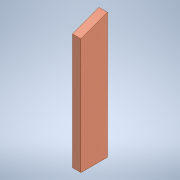
# Autodesk Inventor part: 2x6SupportBracket
Saved by Autodesk Inventor 2022.2 (Build 262287000, 287)
## iProperties
Created: 2021-11-26
Part Number: 2x6SupportBracket
Material: Wood (Walnut)
Document SubType Name: Modeling
Designer: robst
Density: 0.55 g/cm^3
Appearance: Walnut - Natural Polished
Author: robst
Autodesk Inventor part; units mm, degrees
ref_plane "YZ Plane" through (0, 0, 0) normal (1, 0, 0) x (0, 1, 0)
ref_plane "XZ Plane" through (0, 0, 0) normal (0, 1, 0) x (-1, 0, 0)
ref_plane "XY Plane" through (0, 0, 0) normal (0, 0, 1) x (1, 0, 0)
sketch "Sketch4" plane through (0, 0, 0) normal (1, 0, 0) x (0, 1, 0)
  line L0 (0, 0) -> (-609.6, 0)
  line L1 (-609.6, 0) -> (-246.4184, 0)
  line L2 (-609.6, 0) -> (-609.6, -139.7)
  line L3 (-609.6, -139.7) -> (-50.8466, -139.7)
  line L4 (0, 0) -> (50.8466, -139.7)
  line L5 (50.8466, -139.7) -> (-50.8466, -139.7)
  dimension "d12" = 609.6
  dimension "d13" = 139.7
  dimension "d17" = 110
  constraints: 12 end point, 3 horizontal, 1 point on line, 1 vertical
  measures "d12" distance of L0.start L0.end
  measures "d13" distance of L0.end L2.end
  measures "d17" angle of L4 L0
extrude "Extrusion3" add sketch "Sketch4" along normal mid plane 44.45
equation "\"d13\" = depth"
equation "\"d15\" = width"
equation "\"width\" = 44.45"
equation "\"depth\" = 139.7"
body "Solid2"
